simple_spacer (Autodesk Fusion 360 design; units mm, degrees)
Autodesk Fusion 360 part; units mm, degrees
sketch "Sketch" plane through (0, 0, 0) normal (0, 1, 0) x (-1, 0, 0)
  line L0 (30.0004, 1) -> (30.0004, 0)
  line L1 (0.0004, 1) -> (30.0004, 1)
  line L2 (0.0004, 0) -> (0.0004, 1)
  line L3 (30.0004, 0) -> (0.0004, 0)
  line L4 (12, 0) -> (12, -1)
  line L5 (17.9993, -1) -> (17.9993, 0)
  line L6 (17.9993, 0) -> (12, 0)
  line L7 (12, -1) -> (17.9993, -1)
  dimension "d1" = 1
  dimension "d2" = 30
  dimension "d3" = 1
extrude "Extrude2" add sketch "Sketch" along normal blind 1 contours L3 L4 L5 L6 L7 makes body 1
extrude "Extrude1" add sketch "Sketch" along normal blind 9 separate body contours L0 L1 L2 L3 L6 makes body 2
fillet "Fillet3" radius 2 1 edges at (-0.0004, 9, 0.5) on bodies 2
fillet "Fillet4" radius 2 1 edges at (-30.0004, 9, 0.5) on bodies 2
